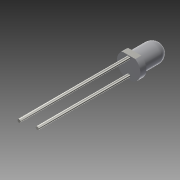
# Autodesk Inventor part: LED
Saved by Autodesk Inventor 2018 (Build 220112000, 112)
## iProperties
Created: 2017-12-07
Part Number: LED
Material: Polycarbonate, Clear
Document SubType Name: Modeling
Designer: Rus
Density: 1.2 g/cm^3
Appearance: Silver
Author: Rus
Autodesk Inventor part; units mm, degrees
ref_plane "YZ Plane" through (0, 0, 0) normal (1, 0, 0) x (0, 1, 0)
ref_plane "XZ Plane" through (0, 0, 0) normal (0, 1, 0) x (-1, 0, 0)
ref_plane "XY Plane" through (0, 0, 0) normal (0, 0, 1) x (1, 0, 0)
sketch "Sketch1" plane through (0, 0, 0) normal (0, 0, 1) x (1, 0, 0)
  line L0 (0, 0) -> (1.925, 0)
  line L1 (1.925, 0) -> (1.925, 1)
  line L2 (1.925, 1) -> (1.5, 1)
  line L3 (1.5, 1) -> (1.5, 3.8)
  line L4 (0, 5.3) -> (0, 5.3)
  line L5 (0, 0) -> (-1.925, 0)
  line L6 (-1.925, 0) -> (-1.925, 1)
  line L7 (-1.925, 1) -> (-1.5, 1)
  line L8 (-1.5, 1) -> (-1.5, 3.8)
  line L9 (0, 5.3) -> (0, 5.3)
  arc A0 (0, 5.3) -> (-1.5, 3.8) centre (0, 3.8) ccw
  arc A1 (1.5, 3.8) -> (0, 5.3) centre (0, 3.8) ccw
  line L10 (0, 5.3) -> (0, 0)
  point P0 (1.5, 5.3)
  dimension "d0" = 1.925
  dimension "d1" = 1
  dimension "d2" = 0.425
  dimension "d3" = 4.3
  dimension "d4" = 1.5
  dimension "d5" = 1.925
  dimension "d6" = 0.425
  dimension "d7" = 1.5
  constraints: 22 end point, 8 perpendicular, 5 point on circle, 4 tangent, 3 point on line, 2 centre point, 2 horizontal, 1 concentric, 1 parallel
  measures "d0" distance of L0.start L0.end
  measures "d1" distance of L0.end L1.end
  measures "d2" distance of L1.end L2.end
  measures "d3" distance of L2.end point (1.5, 5.3)
  measures "d4" distance of point (1.5, 5.3) L4.end
  measures "d5" distance of L0.start L5.end
  measures "d6" distance of L6.end L7.end
  measures "d7" radius of A0
revolve "Revolution1" add sketch "Sketch1" angle 360 about axis through (0, 5.3, 0) along (0, -1, 0) contours L5 L6 L7 L8 A0 L10
sketch "Sketch2" plane through (0, 0, 0) normal (0, -1, 0) x (1, 0, 0)
  circle A0 centre (0, 1.27) radius 0.25
  circle A1 centre (0, -1.27) radius 0.25
  line L0 (0, -1.02) -> (0, 1.02)
  point P0 (0, 0)
  point P1 (0, 0)
  dimension "d10" = 0.5
  dimension "d9" = 2.04
  constraints: 3 vertical, 2 end point, 2 vertical alignment, 1 coincident, 1 midpoint, 4 other
  measures "d9" distance of L0.start L0.end
extrude "Extrusion1" add sketch "Sketch2" along normal blind 18 contours A0
extrude "Extrusion2" add sketch "Sketch2" along normal blind 15 contours A1
sketch "Sketch3" plane through (0, 1, 0) normal (0, 1, 0) x (1, 0, 0)
  circle A0 centre (0, 0) radius 1.5 projected
  circle A1 centre (0, -1.27) radius 0.25 projected
  circle A2 centre (0, 0) radius 1.925 projected
  circle A3 centre (0, 0) radius 1.5 projected
  circle A4 centre (0, 0) radius 1.925 projected
  arc A5 (-1.0778, -1.595) -> (1.0778, -1.595) centre (0, 0) ccw
  line L0 (1.0778, -1.595) -> (-1.0778, -1.595)
  line L1 (0, -1.52) -> (0, -1.595)
  point P0 (0, 0)
  dimension "d17" = 0.075
  constraints: 4 end point, 3 point on circle, 1 centre point, 1 concentric, 1 horizontal, 1 midpoint, 1 perpendicular, 1 vertical alignment, 3 other
  measures "d17" distance of L1.start L1.end
extrude "Extrusion3" cut sketch "Sketch3" against normal up to surface (1 mm away) contours L0 A2 picked at (0.5832, -1.6646)
body "Solid1"
